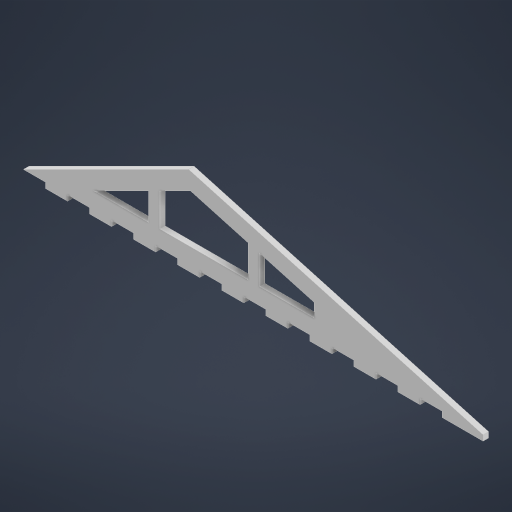
# Autodesk Inventor part: Langbektang houder
Saved by Autodesk Inventor 2023.2 (Build 272271000, 271)
## iProperties
Created: 2020-09-09
Part Number: Langbektang houder
Material: Generic
Document SubType Name: Modeling
Designer: nathan.bollaert
Density: 1 g/cm^3
Appearance: Default
Author: nathan.bollaert
Autodesk Inventor part; units mm, degrees
ref_plane "YZ Plane" through (0, 0, 0) normal (1, 0, 0) x (0, 1, 0)
ref_plane "XZ Plane" through (0, 0, 0) normal (0, 1, 0) x (-1, 0, 0)
ref_plane "XY Plane" through (0, 0, 0) normal (0, 0, 1) x (1, 0, 0)
sketch "Sketch1" plane through (0, 0, 0) normal (0, 0, 1) x (1, 0, 0)
  line L0 (13.8455, -58.3807) -> (313.7199, -67.0622)
  line L1 (313.7199, -67.0622) -> (333.7863, 0)
  line L2 (13.8455, -58.3807) -> (0, 0)
  line L3 (0, 0) -> (333.7863, 0)
  line L4 (120, 60) -> (333.7863, 0)
  line L5 (120, 60) -> (0, 0)
  line L6 (121.2205, 47.1938) -> (50.8328, 12)
  line L7 (211.2205, 12) -> (211.2205, 21.935)
  line L8 (211.2205, 21.935) -> (121.2205, 47.1938)
  line L9 (90.8328, 32) -> (90.8328, 12)
  line L10 (121.2205, 47.1938) -> (124.463, 58.7474)
  line L11 (121.2205, 47.1938) -> (115.8539, 57.927)
  line L12 (211.2205, 12) -> (211.2205, 0)
  line L13 (171.2205, 33.1611) -> (171.2205, 12)
  line L14 (98.8328, 36) -> (98.8328, 12)
  line L15 (90.8328, 12) -> (98.8328, 12)
  line L16 (163.2205, 35.4064) -> (163.2205, 12)
  line L17 (163.2205, 12) -> (171.2205, 12)
  line L18 (211.2205, 12) -> (50.8328, 12)
  dimension "d228" = 105
  dimension "d268" = 60
  dimension "d269" = 70
  dimension "d270" = 300
  dimension "d273" = 120
  dimension "d274" = 60
  dimension "d275" = 105
  dimension "d283" = 90
  dimension "d284" = 40
  dimension "d285" = 40
  dimension "d289" = 8
  dimension "d290" = 12
  constraints: 38 end point, 10 point on line, 3 equal length, 3 horizontal, 3 parallel, 3 perpendicular, 3 vertical, 1 coincident
  measures "d228" angle of L1 L0
  measures "d268" distance of L0.start L3.start
  measures "d269" distance of L0.end L3.end
  measures "d270" distance of L0.start L0.end
  measures "d273" horizontal distance of point (0, 0) L4.start
  measures "d274" vertical distance of point (0, 0) L4.start
  measures "d275" angle of L0 L2
  measures "d283" horizontal distance of L6.start L7.end
  measures "d284" horizontal distance of L7.end L13.start
  measures "d285" horizontal distance of L6.end L9.start
  measures "d289" distance between parallel lines of L9 L14
  measures "d290" distance from line of L3 L6.end
extrude "Extrusion1" add sketch "Sketch1" against normal blind 4 contours L5 L11 L6 L18 L15 L17 L12 L3 | L3 L12 L7 L8 L10 L4 | L5 L4 L10 L11 | L17 L16 L8 L13 | L14 L15 L9 L6
sketch "Sketch2" plane through (0, 0, 0) normal (0, 0, 1) x (1, 0, 0)
  line L0 (0, 0) -> (120, 60) projected
  line L1 (16, 0) -> (16, -4)
  line L2 (16, -4) -> (0, -4)
  line L3 (0, -4) -> (0, 0)
  line L4 (32, 0) -> (48, 0)
  line L5 (48, 0) -> (48, -4)
  line L6 (48, -4) -> (32, -4)
  line L7 (32, -4) -> (32, 0)
  line L8 (64, 0) -> (80, 0)
  line L9 (80, 0) -> (80, -4)
  line L10 (80, -4) -> (64, -4)
  line L11 (64, -4) -> (64, 0)
  line L12 (64, 0) -> (48, 0)
  line L13 (16, 0) -> (32, 0)
  line L14 (0, 0) -> (16, 0)
  line L15 (96, 0) -> (112, 0)
  line L16 (112, 0) -> (112, -4)
  line L17 (112, -4) -> (96, -4)
  line L18 (96, -4) -> (96, 0)
  line L19 (96, 0) -> (80, 0)
  line L20 (160, 0) -> (176, 0)
  line L21 (176, 0) -> (176, -4)
  line L22 (176, -4) -> (160, -4)
  line L23 (160, -4) -> (160, 0)
  line L24 (160, 0) -> (176, 0)
  line L25 (160, 0) -> (176, 0)
  line L26 (176, 0) -> (176, -4)
  line L27 (176, -4) -> (160, -4)
  line L28 (160, -4) -> (160, 0)
  line L29 (160, 0) -> (144, 0)
  line L30 (192, 0) -> (208, 0)
  line L31 (208, 0) -> (208, -4)
  line L32 (208, -4) -> (192, -4)
  line L33 (192, -4) -> (192, 0)
  line L34 (192, 0) -> (176, 0)
  line L35 (224, 0) -> (240, 0)
  line L36 (240, 0) -> (240, -4)
  line L37 (240, -4) -> (224, -4)
  line L38 (224, -4) -> (224, 0)
  line L39 (224, 0) -> (208, 0)
  line L40 (128, 0) -> (144, 0)
  line L41 (144, 0) -> (144, -4)
  line L42 (144, -4) -> (128, -4)
  line L43 (128, -4) -> (128, 0)
  line L44 (128, 0) -> (112, 0)
  line L45 (224, 0) -> (240, 0)
  line L46 (240, 0) -> (240, -4)
  line L47 (240, -4) -> (224, -4)
  line L48 (224, -4) -> (224, 0)
  line L49 (224, 0) -> (240, 0)
  line L50 (256, 0) -> (272, 0)
  line L51 (272, 0) -> (272, -4)
  line L52 (272, -4) -> (256, -4)
  line L53 (256, -4) -> (256, 0)
  line L54 (256, 0) -> (240, 0)
  line L55 (288, 0) -> (304, 0)
  line L56 (304, 0) -> (304, -4)
  line L57 (304, -4) -> (288, -4)
  line L58 (288, -4) -> (288, 0)
  line L59 (288, 0) -> (272, 0)
  line L60 (333.7863, 0) -> (333.7863, -4)
  line L61 (333.7863, 0) -> (0, 0) projected
  line L62 (304, 0) -> (333.7863, 0)
  line L63 (333.7863, -4) -> (0, -4)
  dimension "d292" = 16
  dimension "d296" = 16
  dimension "d297" = 4
  constraints: 122 end point, 32 equal length, 25 perpendicular, 23 parallel, 12 horizontal, 1 coincident, 4 other
  measures "d292" distance of L1.end L2.end
  measures "d296" distance of L1.end L6.end
  measures "d297" distance of L0.start L2.end
extrude "Extrusion2" add sketch "Sketch2" against normal blind 4 contours L13 L7 L63 L1 | L12 L11 L63 L5 | L19 L18 L63 L9 | L44 L43 L63 L16 | L29 L23 L63 L41 | L34 L33 L63 L21 | L39 L38 L63 L31 | L54 L53 L63 L36 | L59 L58 L63 L51 | L61 L60 L63 L56
body "Solid5"
